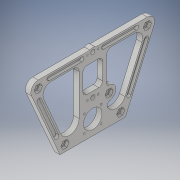
# Autodesk Inventor part: Frame_Stepper
Saved by Autodesk Inventor 2019 (Build 230136000, 136)
## iProperties
Created: 2019-07-29
Part Number: Frame_Stepper
Material: Generic
Document SubType Name: Modeling
Designer: 19879326
Density: 1 g/cm^3
Appearance: Default
Author: 19879326
Autodesk Inventor part; units mm, degrees
ref_plane "YZ Plane" through (0, 0, 0) normal (1, 0, 0) x (0, 1, 0)
ref_plane "XZ Plane" through (0, 0, 0) normal (0, 1, 0) x (-1, 0, 0)
ref_plane "XY Plane" through (0, 0, 0) normal (0, 0, 1) x (1, 0, 0)
sketch "Sketch1" plane through (0, 0, 0) normal (1, 0, 0) x (0, 1, 0)
  line L0 (73.575, 28) -> (65.075, 28)
  line L1 (-73.575, 60) -> (-73.575, -60)
  line L2 (73.575, -28) -> (73.575, 28)
  circle A0 centre (59.575, 0) radius 4
  circle A1 centre (-12.425, 0) radius 4
  circle A2 centre (59.575, 0) radius 7.5
  line L3 (65.075, 28) -> (65.075, 5.099)
  line L4 (65.075, -5.099) -> (65.075, -28)
  circle A3 centre (51.575, -100) radius 4
  circle A4 centre (51.575, 100) radius 4
  arc A5 (65.075, 100) -> (46.1655, 112.3688) centre (51.575, 100) ccw
  arc A6 (46.1655, -112.3688) -> (65.075, -100) centre (51.575, -100) ccw
  line L5 (65.075, 28) -> (65.075, 100)
  line L6 (65.075, -28) -> (65.075, -100)
  line L7 (46.1655, 112.3688) -> (-73.575, 60)
  line L8 (-73.575, -60) -> (46.1655, -112.3688)
  circle A7 centre (-20.425, -30) radius 4
  line L9 (65.075, -28) -> (73.575, -28)
  line L10 (30.0644, 90.0466) -> (-40.7048, 59.0955)
  line L11 (30.0644, -90.0466) -> (-40.7048, -59.0955)
  line L12 (51.075, 76.3035) -> (51.075, 35)
  line L13 (51.075, -76.3035) -> (51.075, -35)
  line L14 (41.075, 25) -> (-33.575, 25)
  line L15 (41.075, -25) -> (-8.9686, -25)
  arc A8 (41.075, 25) -> (51.075, 35) centre (41.075, 35) ccw
  arc A9 (-40.7048, 59.0955) -> (-33.575, 25) centre (-33.575, 42.7932) ccw
  arc A10 (51.075, -35) -> (41.075, -25) centre (41.075, -35) ccw
  circle A11 centre (-20.425, -30) radius 12.5
  line L16 (-31.8814, -25) -> (-33.575, -25)
  arc A12 (-33.575, -25) -> (-40.7048, -59.0955) centre (-33.575, -42.7932) ccw
  circle A13 centre (-61.575, 51.0593) radius 4
  circle A14 centre (-61.575, -51.0593) radius 4
  arc A15 (51.075, 76.3035) -> (30.0644, 90.0466) centre (36.075, 76.3035) ccw
  arc A16 (30.0644, -90.0466) -> (51.075, -76.3035) centre (36.075, -76.3035) ccw
  circle A17 centre (19.575, 0) radius 18
  circle A18 centre (-46.575, 0) radius 17
  circle A19 centre (-62.075, 15.5) radius 1.5
  circle A20 centre (-31.075, 15.5) radius 1.5
  circle A21 centre (-31.075, -15.5) radius 1.5
  circle A22 centre (-62.075, -15.5) radius 1.5
  line L17 (43.575, 18) -> (-2.425, 18)
  line L18 (-2.425, 18) -> (-2.425, -18)
  line L19 (-2.425, -18) -> (43.575, -18)
  line L20 (43.575, -18) -> (43.575, 18)
  point P0 (0, 0)
  point P1 (73.575, 0)
  point P2 (51.075, 58.5072)
  point P3 (51.075, -58.5072)
  point P4 (-20.425, -42.5)
  point P5 (16.0532, -25)
  point P6 (-49.2726, -25)
  point P7 (51.075, 59.4738)
  point P8 (1.575, 0)
  dimension "d1" = 56
  dimension "d2" = 72
  dimension "d3" = 8
  dimension "d4" = 8
  dimension "d5" = 14
  dimension "d13" = 12.425
  dimension "d15" = 15
  dimension "d18" = 5.5
  dimension "d19" = 8
  dimension "d20" = 100
  dimension "d21" = 100
  dimension "d22" = 8
  dimension "d23" = 8
  dimension "d25" = 30
  dimension "d26" = 8
  dimension "d31" = 14
  dimension "d33" = 14
  dimension "d34" = 14
  dimension "d36" = 25
  dimension "d37" = 25
  dimension "d41" = 25
  dimension "d43" = 40
  dimension "d47" = 12
  dimension "d48" = 13
  dimension "d49" = 13
  dimension "d50" = 12
  dimension "d58" = 10
  dimension "d59" = 15
  dimension "d87" = 34
  dimension "d88" = 36
  dimension "d89" = 66.15
  dimension "d90" = 3
  dimension "d91" = 31
  dimension "d92" = 31
  dimension "d93" = 15.5
  dimension "d94" = 15.5
  dimension "d95" = 27
  dimension "d96" = 19.575
  dimension "d97" = 60
  dimension "d98" = 60
  dimension "d142" = 10
  dimension "d143" = 16
  constraints: 42 end point, 23 centre point, 21 point on circle, 15 tangent, 10 equal radius, 9 horizontal alignment, 6 parallel, 6 point on line, 5 horizontal, 5 vertical, 4 coincident, 4 vertical alignment, 2 midpoint, 2 perpendicular
  measures "d1" distance of L2.start L0.start
  measures "d2" distance of A1.centre A0.centre
  measures "d3" diameter of A0
  measures "d4" diameter of A1
  measures "d5" distance from line of L2 A0.centre
  measures "d13" distance of A1.centre point (0, 0)
  measures "d15" diameter of A2
  measures "d18" distance from line of A0.centre L4
  measures "d19" diameter of A4
  measures "d20" vertical distance of A4.centre A0.centre
  measures "d21" vertical distance of A3.centre A0.centre
  measures "d22" horizontal distance of A4.centre A0.centre
  measures "d23" diameter of A7
  measures "d25" vertical distance of A1.centre A7.centre
  measures "d26" horizontal distance of A7.centre A1.centre
  measures "d31" distance between parallel lines of L5 L12
  measures "d33" distance between parallel lines of L7 L10
  measures "d34" distance between parallel lines of L8 L11
  measures "d36" distance from line of L14 A0.centre
  measures "d37" distance from line of A0.centre L15
  measures "d41" diameter of A11
  measures "d43" distance from line of L1 A9.centre
  measures "d47" distance from line of L1 A13.centre
  measures "d48" distance from line of L7 A13.centre
  measures "d49" distance from line of L8 A14.centre
  measures "d50" distance from line of L1 A14.centre
  measures "d58" radius of A8
  measures "d59" radius of A15
  measures "d87" diameter of A18
  measures "d88" diameter of A17
  measures "d89" distance of A18.centre A17.centre
  measures "d90" diameter of A20
  measures "d91" distance of A19.centre A20.centre
  measures "d92" distance of A21.centre A20.centre
  measures "d93" horizontal distance of A18.centre A20.centre
  measures "d94" horizontal distance of A20.centre A18.centre
  measures "d95" distance from line of L1 A18.centre
  measures "d96" distance of point (0, 0) A17.centre
  measures "d97" vertical distance of L1.start A18.centre
  measures "d98" vertical distance of L1.end A18.centre
  measures "d142" distance from line of A1.centre L18
  measures "d143" distance from line of A0.centre L20
extrude "Extrusion3" add sketch "Sketch1" along normal blind 10 contours L3 A2 L4 L6 A6 L8 L1 L7 A5 L5 | A2 | A11
fillet "Fillet1" radius 6 2 edges at (5, -8.9686, -25) (5, -31.8814, -25)
sketch "Sketch3" plane through (10, 0, 0) normal (1, 0, 0) x (0, 0, -1)
  line L0 (-60, -73.575) -> (60, -73.575) projected
  line L1 (-102.0122, 29.9722) -> (-70.0199, -43.1778)
  line L2 (-94.6826, 33.1778) -> (-62.6903, -39.9722)
  line L3 (62.6903, -39.9722) -> (94.6826, 33.1778)
  line L4 (90.0466, 30.0644) -> (59.0955, -40.7048) projected
  line L5 (102.0122, 29.9722) -> (70.0199, -43.1778)
  line L6 (60, -73.575) -> (112.3688, 46.1655) projected
  arc A0 (-94.6826, 33.1778) -> (-102.0122, 29.9722) centre (-98.3474, 31.575) ccw
  arc A1 (-70.0199, -43.1778) -> (-62.6903, -39.9722) centre (-66.3551, -41.575) ccw
  arc A2 (102.0122, 29.9722) -> (94.6826, 33.1778) centre (98.3474, 31.575) ccw
  arc A3 (62.6903, -39.9722) -> (70.0199, -43.1778) centre (66.3551, -41.575) ccw
  line L7 (-59.0955, -40.7048) -> (-90.0466, 30.0644) projected
  line L8 (-112.3688, 46.1655) -> (-60, -73.575) projected
  line L9 (-80, 62.075) -> (-20, 62.075)
  line L10 (-20, 54.075) -> (-80, 54.075)
  line L11 (20, 62.075) -> (80, 62.075)
  line L12 (80, 54.075) -> (20, 54.075)
  arc A4 (-80, 62.075) -> (-80, 54.075) centre (-80, 58.075) ccw
  arc A5 (-20, 54.075) -> (-20, 62.075) centre (-20, 58.075) ccw
  arc A6 (20, 62.075) -> (20, 54.075) centre (20, 58.075) ccw
  arc A7 (80, 54.075) -> (80, 62.075) centre (80, 58.075) ccw
  circle A8 centre (0, 59.575) radius 4 projected
  line L13 (-5.099, 65.075) -> (-100, 65.075) projected
  line L14 (-76.3035, 51.075) -> (-35, 51.075) projected
  line L15 (35, 51.075) -> (76.3035, 51.075) projected
  line L16 (100, 65.075) -> (5.099, 65.075) projected
  circle A9 centre (-51.0593, -61.575) radius 4
  circle A10 centre (-51.0593, -61.575) radius 4 projected
  circle A11 centre (-100, 51.575) radius 4
  circle A12 centre (100, 51.575) radius 4
  circle A13 centre (-100, 51.575) radius 4 projected
  circle A14 centre (100, 51.575) radius 4 projected
  point P0 (0, 0)
  dimension "d71" = 3
  dimension "d72" = 3
  dimension "d73" = 3
  dimension "d74" = 3
  dimension "d78" = 20
  dimension "d79" = 20
  dimension "d81" = 3
  dimension "d82" = 3
  dimension "d83" = 3
  dimension "d84" = 3
  dimension "d145" = 20
  dimension "d146" = 20
  dimension "d147" = 20
  dimension "d148" = 20
  constraints: 16 end point, 16 point on circle, 16 tangent, 11 centre point, 7 parallel, 3 concentric, 3 equal radius, 2 horizontal, 2 horizontal alignment
  measures "d71" distance between parallel lines of L7 L2
  measures "d72" distance between parallel lines of L8 L1
  measures "d73" distance between parallel lines of L6 L5
  measures "d74" distance between parallel lines of L4 L3
  measures "d78" horizontal distance of A8.centre A5.centre
  measures "d79" horizontal distance of A6.centre A8.centre
  measures "d81" distance between parallel lines of L13 L9
  measures "d82" distance between parallel lines of L14 L10
  measures "d83" distance between parallel lines of L15 L12
  measures "d84" distance between parallel lines of L16 L11
  measures "d145" vertical distance of A9.centre A1.centre
  measures "d146" horizontal distance of A11.centre A4.centre
  measures "d147" vertical distance of A0.centre A11.centre
  measures "d148" horizontal distance of A7.centre A12.centre
extrude "Extrusion5" cut sketch "Sketch3" against normal blind 5 contours A0 L2 A1 L1 | L3 A2 L5 A3 | L9 A5 L10 A4 | L11 A7 L12 A6
sketch "Sketch4" plane through (10, 0, 0) normal (1, 0, 0) x (0, 0, -1)
  line L0 (-103.7528, 58.075) -> (-96.2472, 58.075)
  line L1 (-96.2472, 58.075) -> (-92.4944, 51.575)
  line L2 (-92.4944, 51.575) -> (-96.2472, 45.075)
  line L3 (-96.2472, 45.075) -> (-103.7528, 45.075)
  line L4 (-103.7528, 45.075) -> (-107.5056, 51.575)
  line L5 (-107.5056, 51.575) -> (-103.7528, 58.075)
  circle A0 centre (-100, 51.575) radius 6.5
  circle A1 centre (-100, 51.575) radius 4
  line L6 (96.2472, 58.075) -> (103.7528, 58.075)
  line L7 (103.7528, 58.075) -> (107.5056, 51.575)
  line L8 (107.5056, 51.575) -> (103.7528, 45.075)
  line L9 (103.7528, 45.075) -> (96.2472, 45.075)
  line L10 (96.2472, 45.075) -> (92.4944, 51.575)
  line L11 (92.4944, 51.575) -> (96.2472, 58.075)
  circle A2 centre (100, 51.575) radius 6.5
  circle A3 centre (100, 51.575) radius 4
  circle A4 centre (100, 51.575) radius 4
  line L12 (-47.3065, -55.075) -> (-43.5537, -61.575)
  line L13 (-43.5537, -61.575) -> (-47.3065, -68.075)
  line L14 (-47.3065, -68.075) -> (-54.8121, -68.075)
  circle A5 centre (-51.0593, -61.575) radius 4
  circle A6 centre (-51.0593, -61.575) radius 6.5
  line L15 (-54.8121, -68.075) -> (-58.5648, -61.575)
  line L16 (-58.5648, -61.575) -> (-54.8121, -55.075)
  line L17 (-54.8121, -55.075) -> (-47.3065, -55.075)
  circle A7 centre (-51.0593, -61.575) radius 4
  line L18 (54.8121, -68.075) -> (47.3065, -68.075)
  line L19 (58.5648, -61.575) -> (54.8121, -68.075)
  line L20 (47.3065, -68.075) -> (43.5537, -61.575)
  circle A8 centre (51.0593, -61.575) radius 4
  line L21 (43.5537, -61.575) -> (47.3065, -55.075)
  circle A9 centre (51.0593, -61.575) radius 6.5
  line L22 (47.3065, -55.075) -> (54.8121, -55.075)
  line L23 (54.8121, -55.075) -> (58.5648, -61.575)
  circle A10 centre (51.0593, -61.575) radius 4
  circle A11 centre (-100, 51.575) radius 4
  circle A12 centre (-51.0593, -61.575) radius 4
  circle A13 centre (51.0593, -61.575) radius 4
  circle A14 centre (100, 51.575) radius 4
  line L24 (26.2472, -13.925) -> (33.7528, -13.925)
  line L25 (33.7528, -13.925) -> (37.5056, -20.425)
  line L26 (37.5056, -20.425) -> (33.7528, -26.925)
  line L27 (33.7528, -26.925) -> (26.2472, -26.925)
  line L28 (26.2472, -26.925) -> (22.4944, -20.425)
  line L29 (22.4944, -20.425) -> (26.2472, -13.925)
  circle A15 centre (30, -20.425) radius 6.5
  circle A16 centre (30, -20.425) radius 4
  circle A17 centre (30, -20.425) radius 4
  circle A18 centre (30, -20.425) radius 4 projected
  circle A19 centre (-51.0593, -61.575) radius 4 projected
  circle A20 centre (51.0593, -61.575) radius 4 projected
  circle A21 centre (100, 51.575) radius 4 projected
  circle A22 centre (-100, 51.575) radius 4 projected
  point P0 (0, 0)
  point P1 (0, 0)
  dimension "d132" = 13
  dimension "d133" = 13
  dimension "d134" = 13
  dimension "d135" = 13
  dimension "d136" = 8
  dimension "d137" = 8
  dimension "d138" = 8
  dimension "d139" = 8
  dimension "d140" = 13
  dimension "d141" = 8
  constraints: 60 end point, 30 tangent, 21 concentric, 20 equal length, 18 centre point, 5 horizontal, 5 parallel
  measures "d132" diameter of A0
  measures "d133" diameter of A2
  measures "d134" diameter of A6
  measures "d135" diameter of A9
  measures "d136" diameter of A1
  measures "d137" diameter of A3
  measures "d138" diameter of A8
  measures "d139" diameter of A5
  measures "d140" diameter of A15
  measures "d141" diameter of A16
extrude "Extrusion6" cut sketch "Sketch4" against normal blind 5
fillet "Fillet2" radius 7 4 edges at (5, -2.425, 18) (5, 43.575, 18) (5, 43.575, -18) (5, -2.425, -18)
sketch "Sketch5" plane through (10, 0, 0) normal (1, 0, 0) x (0, 0, -1)
  circle A0 centre (-10, 59.575) radius 1.5
  circle A1 centre (10, 59.575) radius 1.5
  circle A2 centre (0, 59.575) radius 4
  circle A3 centre (0, 59.575) radius 4 projected
  circle A4 centre (-10, -12.425) radius 1.5
  circle A5 centre (10, -12.425) radius 1.5
  circle A6 centre (0, -12.425) radius 4
  circle A7 centre (0, -12.425) radius 4
  circle A8 centre (0, -12.425) radius 4 projected
  point P0 (0, 0)
  dimension "d149" = 3
  dimension "d150" = 10
  dimension "d151" = 10
  dimension "d154" = 3
  dimension "d155" = 10
  dimension "d156" = 10
  constraints: 7 centre point, 5 equal radius, 4 horizontal alignment, 3 concentric
  measures "d149" diameter of A0
  measures "d150" distance of A2.centre A0.centre
  measures "d151" distance of A1.centre A2.centre
  measures "d154" diameter of A4
  measures "d155" distance of A6.centre A4.centre
  measures "d156" distance of A5.centre A6.centre
extrude "Extrusion7" cut sketch "Sketch5" against normal blind 10 contours A0 | A1 | A4 | A5
body "Solid3"
